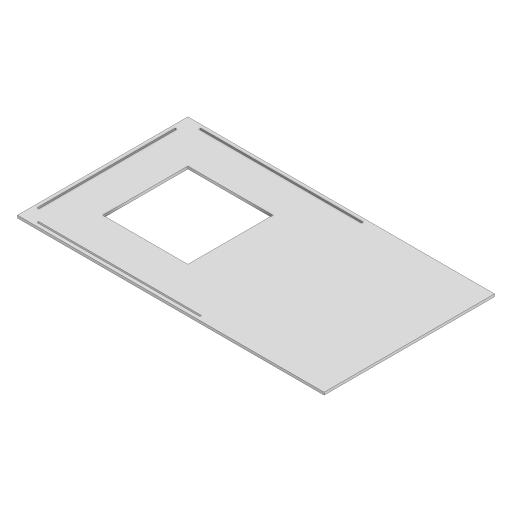
# Autodesk Inventor part: BottomPlateRS3
Saved by Autodesk Inventor 2024.3 (Build 283343000, 343)
## iProperties
Created: 2025-06-13
Part Number: BottomPlateRS3
Material: Steel
Document SubType Name: Modeling
Designer: ajclo
Density: 7.85 g/cm^3
Appearance: Plate
Mass: 1460.1 g
Surface Area: 1285.6 cm^2
Volume: 186 cm^3
Author: ajclo
Autodesk Inventor part; units mm, degrees
ref_plane "YZ Plane" through (0, 0, 0) normal (1, 0, 0) x (0, 1, 0)
ref_plane "XZ Plane" through (0, 0, 0) normal (0, 1, 0) x (-1, 0, 0)
ref_plane "XY Plane" through (0, 0, 0) normal (0, 0, 1) x (1, 0, 0)
sketch "Sketch1" plane through (0, 0, 0) normal (0, 1, 0) x (-1, 0, 0)
  line L0 (50, 50) -> (-50, 50)
  line L1 (-50, 50) -> (-50, -50)
  line L2 (-50, -50) -> (50, -50)
  line L3 (50, -50) -> (50, 50)
  line L4 (50, 50) -> (-50, -50) construction
  line L5 (-50, 50) -> (50, -50) construction
  line L6 (100, 100) -> (-100, 100)
  line L7 (-100, 100) -> (-100, -100)
  line L8 (-100, -100) -> (100, -100)
  line L9 (100, -100) -> (100, 100)
  line L10 (100, 100) -> (-100, -100) construction
  line L11 (-100, 100) -> (100, -100) construction
  line L12 (-50, 100) -> (-260, 100)
  line L13 (-260, 100) -> (-260, -100)
  line L14 (-260, -100) -> (-50, -100)
  line L15 (-50, -100) -> (-50, 100)
  point P0 (0, 0)
  dimension "d0" = 100
  dimension "d1" = 100
  dimension "d2" = 200
  dimension "d3" = 50
  dimension "d4" = 210
  dimension "d5" = 0
  dimension "d6" = 200
  constraints: 32 end point, 6 parallel, 4 midpoint, 3 horizontal, 3 perpendicular, 1 point on line
  measures "d0" distance of L1.end L2.end
  measures "d1" distance of L2.end L0.start
  measures "d2" distance of L8.end L6.start
  measures "d3" distance between parallel lines of L3 L9
  measures "d4" distance between parallel lines of L13 L1
  measures "d5" distance between parallel lines of L1 L15
  measures "d6" distance between parallel lines of L12 L14
extrude "Extrusion1" add sketch "Sketch1" along normal blind 3 contours L0 L15 L6 L9 L8 L2 L3 | L1 L15 L8 L7 L6 | L7 L14 L13 L12
sketch "Sketch3" plane through (0, 0, 0) normal (0, -1, 0) x (1, 0, 0)
  line L0 (110, 96) -> (-96, 96)
  line L1 (-96, 96) -> (-96, -96)
  line L2 (-96, -96) -> (110, -96)
  line L3 (110, -96) -> (110, 96)
  line L4 (-94, -94) -> (108, -94)
  line L5 (108, -94) -> (108, 94)
  line L6 (108, 94) -> (-94, 94)
  line L7 (-94, 94) -> (-94, -94)
  line L8 (-100, -100) -> (-100, 100) projected
  line L9 (260, -100) -> (-100, -100) projected
  line L10 (-100, 100) -> (260, 100) projected
  line L11 (260, 100) -> (260, -100) projected
  line L12 (108, 94) -> (110, 94)
  line L13 (108, -94) -> (110, -94)
  line L14 (-96, 96) -> (-81, 96)
  line L15 (-81, 96) -> (-81, 81)
  line L16 (-81, 81) -> (-96, 81)
  line L17 (-96, 81) -> (-96, 96)
  line L18 (-96, -96) -> (-81, -96)
  line L19 (-81, -96) -> (-81, -81)
  line L20 (-81, -81) -> (-96, -81)
  line L21 (-96, -81) -> (-96, -96)
  point P0 (0, 0)
  point P1 (-81, -94)
  point P2 (-94, -81)
  point P3 (-94, 81)
  point P4 (-81, 94)
  dimension "d13" = 2
  dimension "d14" = 2
  dimension "d15" = 4
  dimension "d16" = 4
  dimension "d17" = 4
  dimension "d18" = 2
  dimension "d19" = 150
  dimension "d20" = 2
  dimension "d21" = 15
  dimension "d22" = 15
  dimension "d23" = 15
  dimension "d24" = 15
  constraints: 36 end point, 8 parallel, 5 horizontal, 5 perpendicular, 3 point on line
  measures "d13" distance between parallel lines of L6 L0
  measures "d14" distance between parallel lines of L1 L7
  measures "d15" distance between parallel lines of L8 L1
  measures "d16" distance between parallel lines of L9 L2
  measures "d17" distance between parallel lines of L10 L0
  measures "d18" distance between parallel lines of L2 L4
  measures "d19" distance between parallel lines of L11 L3
  measures "d20" distance between parallel lines of L3 L5
  measures "d21" distance of L14.end L15.end
  measures "d22" distance of L15.end L16.end
  measures "d23" distance of L19.end L20.end
  measures "d24" distance of L18.end L19.end
extrude "Extrusion3" cut sketch "Sketch3" against normal blind 10 contours L3 L12 L6 L15 L0 | L3 L2 L19 L4 L13 | L16 L7 L20 L1
equation "\"d14\" = d13"
equation "\"d18\" = d13"
equation "\"d20\" = d14"
equation "\"d24\" = d21"
body "Solid1"
